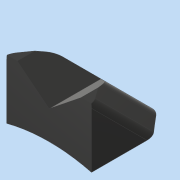
# Autodesk Inventor part: RearMount
Saved by Autodesk Inventor 2017.3 (Build 213256000, 256)
## iProperties
Created: 2018-08-31
Part Number: RearMount
Material: ABS Plastic
Document SubType Name: Modeling
Designer: Derek Wider
Density: 1.06 g/cm^3
Appearance: Smooth - Black
Author: Derek Wider
Autodesk Inventor part; units mm, degrees
ref_plane "YZ Plane" through (0, 0, 0) normal (1, 0, 0) x (0, 1, 0)
ref_plane "XZ Plane" through (0, 0, 0) normal (0, 1, 0) x (-1, 0, 0)
ref_plane "XY Plane" through (0, 0, 0) normal (0, 0, 1) x (1, 0, 0)
sketch "Sketch1" plane through (0, 0, 0) normal (0, 0, 1) x (1, 0, 0)
  line L0 (0, 0) -> (0, 17.78)
  line L1 (25.4, 17.78) -> (25.4, 0)
  arc A0 (25.4, 0) -> (0, 0) centre (12.7, -49.1869) ccw
  line L2 (0, 17.78) -> (3.175, 17.78)
  line L3 (3.175, 17.78) -> (12.7, 10.16)
  line L4 (12.7, 10.16) -> (22.225, 17.78)
  line L5 (22.225, 17.78) -> (25.4, 17.78)
  dimension "d4" = 17.78
  dimension "d5" = 25.4
  dimension "d6" = 101.6
  dimension "d7" = 3.175
  dimension "d8" = 7.62
  constraints: 12 end point, 2 equal length, 2 horizontal alignment, 2 point on circle, 1 centre point, 1 horizontal, 1 perpendicular, 1 point on line, 1 vertical
  measures "d4" distance of L0.start L0.end
  measures "d5" distance of L0.end L1.start
  measures "d6" diameter of A0
  measures "d7" distance of L4.end L1.start
  measures "d8" vertical distance of L3.end L4.end
extrude "Extrusion1" add sketch "Sketch1" along normal blind 25.4
chamfer "Chamfer1" distance 17.526 angle 45 2 edges at (23.8125, 17.78, 0) (1.5875, 17.78, 0)
chamfer "Chamfer2" distance 5.08 angle 45 2 edges at (25.4, 9.017, 8.763) (0, 9.017, 8.763)
fillet "Fillet1" radius 3.175 4 edges at (25.4, 8.89, 15.8202) (20.32, 8.6472, 8.3932) (5.08, 8.6472, 8.3932) (0, 8.89, 15.8202)
body "Solid1"
